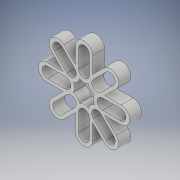
# Autodesk Inventor part: location hole mounter
Saved by Autodesk Inventor 2019 (Build 230136000, 136)
## iProperties
Created: 2018-10-02
Part Number: location hole mounter
Material: Generic
Document SubType Name: Modeling
Designer: HIVE
Density: 1 g/cm^3
Appearance: Default
Author: HIVE
Autodesk Inventor part; units mm, degrees
ref_plane "YZ Plane" through (0, 0, 0) normal (1, 0, 0) x (0, 1, 0)
ref_plane "XZ Plane" through (0, 0, 0) normal (0, 1, 0) x (-1, 0, 0)
ref_plane "XY Plane" through (0, 0, 0) normal (0, 0, 1) x (1, 0, 0)
sketch "Sketch1" plane through (0, 0, 0) normal (0, 0, 1) x (1, 0, 0)
  line L0 (0, 30.4699) -> (0, 15.4699) construction
  line L1 (4, 30.4699) -> (4, 15.4699)
  line L2 (-4, 15.4699) -> (-4, 30.4699)
  arc A0 (4, 30.4699) -> (-4, 30.4699) centre (0, 30.4699) ccw
  arc A1 (-4, 15.4699) -> (4, 15.4699) centre (0, 15.4699) ccw
  circle A2 centre (0, 0) radius 22.9699 construction
  arc A3 (-18.717, 24.3739) -> (-24.3739, 18.717) centre (-21.5455, 21.5455) ccw
  line L3 (-18.717, 24.3739) -> (-8.1104, 13.7673)
  arc A4 (-13.7673, 8.1104) -> (-8.1104, 13.7673) centre (-10.9389, 10.9389) ccw
  line L4 (-13.7673, 8.1104) -> (-24.3739, 18.717)
  circle A5 centre (0, 0) radius 22.9699 construction
  arc A6 (-30.4699, 4) -> (-30.4699, -4) centre (-30.4699, 0) ccw
  line L5 (-30.4699, 4) -> (-15.4699, 4)
  arc A7 (-15.4699, -4) -> (-15.4699, 4) centre (-15.4699, 0) ccw
  line L6 (-15.4699, -4) -> (-30.4699, -4)
  circle A8 centre (0, 0) radius 22.9699 construction
  arc A9 (-24.3739, -18.7171) -> (-18.717, -24.3739) centre (-21.5455, -21.5455) ccw
  line L7 (-24.3739, -18.7171) -> (-13.7673, -8.1105)
  arc A10 (-8.1104, -13.7673) -> (-13.7673, -8.1105) centre (-10.9389, -10.9389) ccw
  line L8 (-8.1104, -13.7673) -> (-18.717, -24.3739)
  circle A11 centre (0, 0) radius 22.9699 construction
  arc A12 (-4, -30.4699) -> (4, -30.4699) centre (0, -30.4699) ccw
  line L9 (-4, -30.4699) -> (-4, -15.4699)
  arc A13 (4, -15.4699) -> (-4, -15.4699) centre (0, -15.4699) ccw
  line L10 (4, -15.4699) -> (4, -30.4699)
  circle A14 centre (0, 0) radius 22.9699 construction
  arc A15 (18.717, -24.3739) -> (24.3739, -18.7171) centre (21.5455, -21.5455) ccw
  line L11 (18.717, -24.3739) -> (8.1104, -13.7673)
  arc A16 (13.7673, -8.1105) -> (8.1104, -13.7673) centre (10.9389, -10.9389) ccw
  line L12 (13.7673, -8.1105) -> (24.3739, -18.7171)
  circle A17 centre (0, 0) radius 22.9699 construction
  arc A18 (30.4699, -4) -> (30.4699, 4) centre (30.4699, 0) ccw
  line L13 (30.4699, -4) -> (15.4699, -4)
  arc A19 (15.4699, 4) -> (15.4699, -4) centre (15.4699, 0) ccw
  line L14 (15.4699, 4) -> (30.4699, 4)
  circle A20 centre (0, 0) radius 22.9699 construction
  arc A21 (24.3739, 18.717) -> (18.717, 24.3739) centre (21.5455, 21.5455) ccw
  line L15 (24.3739, 18.717) -> (13.7673, 8.1104)
  arc A22 (8.1104, 13.7673) -> (13.7673, 8.1104) centre (10.9389, 10.9389) ccw
  line L16 (8.1104, 13.7673) -> (18.717, 24.3739)
  circle A23 centre (0, 0) radius 22.9699 construction
  line L17 (18.3635, 24.7274) -> (7.7569, 14.1208)
  arc A24 (7.7569, 14.1208) -> (14.1208, 7.7569) centre (10.9389, 10.9389) ccw
  line L18 (14.1208, 7.7569) -> (24.7275, 18.3635)
  arc A25 (24.7275, 18.3635) -> (18.3635, 24.7274) centre (21.5455, 21.5455) ccw
  line L19 (-4.5, 30.4699) -> (-4.5, 15.4699)
  arc A26 (-4.5, 15.4699) -> (4.5, 15.4699) centre (0, 15.4699) ccw
  line L20 (4.5, 15.4699) -> (4.5, 30.4699)
  arc A27 (4.5, 30.4699) -> (-4.5, 30.4699) centre (0, 30.4699) ccw
  line L21 (-7.7569, 14.1208) -> (-18.3635, 24.7274)
  arc A28 (-18.3635, 24.7274) -> (-24.7275, 18.3635) centre (-21.5455, 21.5455) ccw
  line L22 (-24.7275, 18.3635) -> (-14.1208, 7.7569)
  arc A29 (-14.1208, 7.7569) -> (-7.7569, 14.1208) centre (-10.9389, 10.9389) ccw
  line L23 (-15.4699, 4.5) -> (-30.4699, 4.5)
  arc A30 (-30.4699, 4.5) -> (-30.4699, -4.5) centre (-30.4699, 0) ccw
  line L24 (-30.4699, -4.5) -> (-15.4699, -4.5)
  arc A31 (-15.4699, -4.5) -> (-15.4699, 4.5) centre (-15.4699, 0) ccw
  line L25 (15.4699, -4.5) -> (30.4699, -4.5)
  arc A32 (30.4699, -4.5) -> (30.4699, 4.5) centre (30.4699, 0) ccw
  line L26 (30.4699, 4.5) -> (15.4699, 4.5)
  arc A33 (15.4699, 4.5) -> (15.4699, -4.5) centre (15.4699, 0) ccw
  line L27 (-14.1209, -7.7569) -> (-24.7275, -18.3635)
  arc A34 (-24.7275, -18.3635) -> (-18.3635, -24.7275) centre (-21.5455, -21.5455) ccw
  line L28 (-18.3635, -24.7275) -> (-7.7569, -14.1209)
  arc A35 (-7.7569, -14.1209) -> (-14.1209, -7.7569) centre (-10.9389, -10.9389) ccw
  line L29 (-4.5, -15.4699) -> (-4.5, -30.4699)
  arc A36 (-4.5, -30.4699) -> (4.5, -30.4699) centre (0, -30.4699) ccw
  line L30 (4.5, -30.4699) -> (4.5, -15.4699)
  arc A37 (4.5, -15.4699) -> (-4.5, -15.4699) centre (0, -15.4699) ccw
  line L31 (7.7569, -14.1209) -> (18.3635, -24.7275)
  arc A38 (18.3635, -24.7275) -> (24.7275, -18.3635) centre (21.5455, -21.5455) ccw
  line L32 (24.7275, -18.3635) -> (14.1208, -7.7569)
  arc A39 (14.1208, -7.7569) -> (7.7569, -14.1209) centre (10.9389, -10.9389) ccw
  circle A40 centre (0, 0) radius 9
  line L33 (0, 30.9133) -> (0, 15.0265) construction
  line L34 (-7.1776, 30.9133) -> (-7.1776, 15.0265)
  line L35 (7.1776, 15.0265) -> (7.1776, 30.9133)
  arc A41 (7.1776, 30.9133) -> (-7.1776, 30.9133) centre (0, 30.9133) ccw
  arc A42 (-7.1776, 15.0265) -> (7.1776, 15.0265) centre (0, 15.0265) ccw
  arc A43 (-16.7836, 26.9344) -> (-26.9344, 16.7836) centre (-21.859, 21.859) ccw
  line L36 (-5.55, 15.7007) -> (-16.7836, 26.9344)
  arc A44 (-15.7007, 5.5499) -> (-5.55, 15.7007) centre (-10.6253, 10.6253) ccw
  line L37 (-26.9344, 16.7836) -> (-15.7007, 5.5499)
  arc A45 (-30.9133, 7.1776) -> (-30.9133, -7.1777) centre (-30.9133, 0) ccw
  line L38 (-15.0265, 7.1776) -> (-30.9133, 7.1776)
  arc A46 (-15.0265, -7.1777) -> (-15.0265, 7.1776) centre (-15.0265, 0) ccw
  line L39 (-30.9133, -7.1777) -> (-15.0265, -7.1777)
  arc A47 (-26.9344, -16.7837) -> (-16.7836, -26.9344) centre (-21.859, -21.859) ccw
  line L40 (-15.7007, -5.55) -> (-26.9344, -16.7837)
  arc A48 (-5.55, -15.7007) -> (-15.7007, -5.55) centre (-10.6253, -10.6253) ccw
  line L41 (-16.7836, -26.9344) -> (-5.55, -15.7007)
  arc A49 (-7.1776, -30.9133) -> (7.1776, -30.9133) centre (0, -30.9133) ccw
  line L42 (-7.1776, -15.0265) -> (-7.1776, -30.9133)
  arc A50 (7.1776, -15.0265) -> (-7.1776, -15.0265) centre (0, -15.0265) ccw
  line L43 (7.1776, -30.9133) -> (7.1776, -15.0265)
  arc A51 (16.7836, -26.9344) -> (26.9344, -16.7837) centre (21.859, -21.859) ccw
  line L44 (5.55, -15.7007) -> (16.7836, -26.9344)
  arc A52 (15.7007, -5.55) -> (5.55, -15.7007) centre (10.6253, -10.6253) ccw
  line L45 (26.9344, -16.7837) -> (15.7007, -5.55)
  arc A53 (30.9133, -7.1777) -> (30.9133, 7.1776) centre (30.9133, 0) ccw
  line L46 (15.0265, -7.1777) -> (30.9133, -7.1777)
  arc A54 (15.0265, 7.1776) -> (15.0265, -7.1777) centre (15.0265, 0) ccw
  line L47 (30.9133, 7.1776) -> (15.0265, 7.1776)
  arc A55 (26.9344, 16.7836) -> (16.7836, 26.9344) centre (21.859, 21.859) ccw
  line L48 (15.7007, 5.5499) -> (26.9344, 16.7836)
  arc A56 (5.55, 15.7007) -> (15.7007, 5.5499) centre (10.6253, 10.6253) ccw
  line L49 (16.7836, 26.9344) -> (5.55, 15.7007)
  point P0 (0, 0)
  point P1 (0, 22.9699)
  point P2 (-16.2422, 16.2422)
  point P3 (-22.9699, 0)
  point P4 (-16.2422, -16.2422)
  point P5 (0, -22.9699)
  point P6 (16.2422, -16.2422)
  point P7 (22.9699, 0)
  point P8 (16.2422, 16.2422)
  dimension "d2" = 4
  dimension "d3" = 15
  dimension "d4" = 360
  dimension "d6" = 0.5
  dimension "d7" = 0.5
  dimension "d8" = 0.5
  dimension "d9" = 0.5
  dimension "d10" = 0.5
  dimension "d11" = 0.5
  dimension "d12" = 0.5
  dimension "d13" = 0.5
  dimension "d14" = 18
  dimension "d17" = 360
  constraints: 104 end point, 96 point on circle, 49 centre point, 9 tangent, 4 coincident, 3 parallel, 2 horizontal alignment, 2 midpoint, 2 vertical alignment, 1 point on line, 1 vertical, 228 other
  measures "d2" radius of A1
  measures "d3" distance of L0.start L0.end
  measures "d6" distance between parallel lines of L16 L17
  measures "d7" radial gap between concentric circles of A0 A27
  measures "d8" distance between parallel lines of L3 L21
  measures "d9" radial gap between concentric circles of A7 A31
  measures "d10" radial gap between concentric circles of A19 A33
  measures "d11" radial gap between concentric circles of A10 A35
  measures "d12" radial gap between concentric circles of A13 A37
  measures "d13" radial gap between concentric circles of A16 A39
  measures "d14" diameter of A40
extrude "Extrusion1" add sketch "Sketch1" along normal blind 10 contours L17 A24 A42 L35 L49 A55 L48 L47 A54 L18 A25 | A24 A54 A56 A40 A42 | A42 A56 L49 L35 | A54 L47 L48 A56 | A42 A40 A44 A26 A56 | A56 A33 A52 A54 A40 | A42 A40 | A26 L20 A27 L19 A44 L36 L34 A41 L35 L49 A56 | A40 A56 | L47 A53 L46 L45 A52 A33 L25 A32 L26 A56 L48 | A40 A54 | A44 A42 L34 L36 | A52 L45 L46 A54 | A44 A40 | A40 A44 A46 A29 A42 | A52 A54 A39 A50 A40 | A40 A52 | A29 L21 A28 L22 A46 L38 L37 A43 L36 L34 A42 | L45 A51 L44 L43 A50 A39 L31 A38 L32 A54 L46 | A46 A40 | A40 A46 A48 A31 A44 | A44 L37 L38 A46 | A50 A52 A37 A48 A40 | A40 A50 | A50 L43 L44 A52 | A31 L23 A30 L24 A48 L40 L39 A45 L38 L37 A44 | A52 L44 L43 A49 L42 L41 A48 A37 L29 A36 L30 | A48 A40 | A40 A48 A50 A35 A46 | A46 L39 L40 A48 | A48 L41 L42 A50 | A35 L27 A34 L28 A50 L42 L41 A47 L40 L39 A46
body "Solid1"
